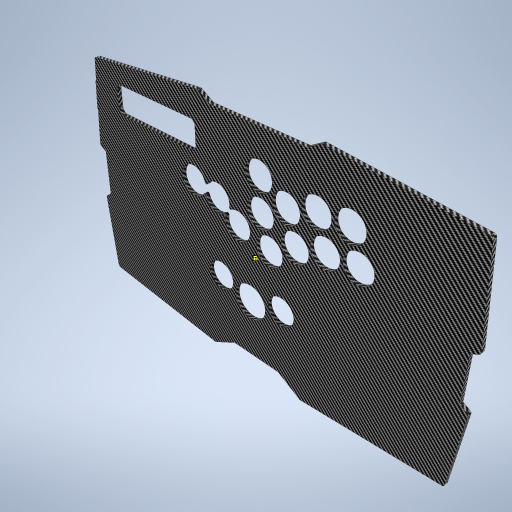
# Autodesk Inventor part: Top_Plate
Saved by Autodesk Inventor 2024 (Build 280153000, 153)
## iProperties
Created: 2023-09-20
Part Number: Top_Plate
Material: 常规
Document SubType Name: Modeling
Designer: nicx5
Density: 1 g/cm^3
Appearance: 碳纤维
Author: nicx5
Autodesk Inventor part; units mm, degrees
ref_plane "YZ Plane" through (0, 0, 0) normal (1, 0, 0) x (0, 1, 0)
ref_plane "XZ Plane" through (0, 0, 0) normal (0, 1, 0) x (-1, 0, 0)
derived "Frame.ipt"
sketch "top面板草图" plane through (0, 0, -3) normal (0, 0, 1) x (1, 0, 0)
  line L0 (-129.5, 55) -> (-52.5, 55)
  line L1 (-52.5, 55) -> (-52.5, 76.5)
  line L2 (-129.5, 76.5) -> (-52.5, 76.5)
  line L3 (-129.5, 55) -> (-129.5, 76.5)
  circle A0 centre (-55.7514, 33.4183) radius 11.5
  circle A1 centre (-34.0856, 29.598) radius 11.5
  circle A2 centre (-16.0643, 16.9793) radius 11.5
  circle A3 centre (-32.1234, -29.7121) radius 11.5
  circle A4 centre (-5.0643, -36.9094) radius 14.5
  circle A5 centre (21.9949, -29.7121) radius 11.5
  circle A6 centre (11.4783, 10.9768) radius 11.5
  circle A7 centre (3.7009, 34.6338) radius 11.5
  circle A8 centre (2.0127, 59.4994) radius 11.5
  circle A9 centre (24.0951, 47.2859) radius 11.5
  circle A10 centre (31.8725, 23.629) radius 11.5
  circle A11 centre (54.6939, 31.0574) radius 11.5
  circle A12 centre (46.9166, 54.7144) radius 11.5
  circle A13 centre (70.8507, 56.4914) radius 11.5
  circle A14 centre (78.628, 32.8344) radius 11.5
  line L4 (157.6336, 21.2378) -> (151.7356, 88.6532)
  line L5 (151.7356, 88.6532) -> (48.367, 97.6967)
  line L6 (48.367, 97.6967) -> (38.067, 91.75)
  line L7 (38.067, 91.75) -> (-38.067, 91.75)
  line L8 (-38.067, 91.75) -> (-48.367, 97.6967)
  line L9 (-48.367, 97.6967) -> (-151.7356, 88.6532)
  line L10 (-151.7356, 88.6532) -> (-153.2586, 71.2446)
  line L11 (-153.2586, 71.2446) -> (-154.5006, 70.2025)
  line L12 (157.6336, 21.2378) -> (151.75, 17.8409)
  line L13 (151.75, -17.8409) -> (157.6336, -21.2378)
  line L14 (157.6336, -21.2378) -> (152.1781, -83.5953)
  line L15 (-20.7465, -81.75) -> (20.7465, -81.75)
  line L16 (20.7465, -81.75) -> (40.8177, -93.3381)
  line L17 (40.8177, -93.3381) -> (152.1781, -83.5953)
  line L18 (-157.6336, -21.2378) -> (-152.1781, -83.5953)
  line L19 (-152.1781, -83.5953) -> (-40.8177, -93.3381)
  line L20 (-40.8177, -93.3381) -> (-20.7465, -81.75)
  line L21 (-157.6336, -21.2378) -> (-151.7501, -17.841)
  line L22 (-151.7501, 17.841) -> (-157.6336, 21.2378)
  line L23 (-157.6336, 21.2378) -> (-155.158, 49.5347)
  line L24 (-155.158, 49.5347) -> (-156.2001, 50.7767)
  line L25 (-154.5006, 70.2025) -> (-155.6, 70.2986)
  line L26 (-156.2001, 50.7767) -> (-157.2995, 50.8728)
  line L27 (-155.6, 70.2986) -> (-157.2995, 50.8728)
  line L28 (-151.7501, -17.841) -> (-151.7501, 17.841)
  line L29 (151.75, 17.8409) -> (151.75, -17.8409)
  point P0 (0, 0)
  point P1 (-154.577, 70.4647)
  point P2 (-156.3209, 50.5317)
  point P3 (-26.9988, 20.5412)
  point P4 (-45.5009, 28.205)
  point P5 (-44.3361, 34.8113)
  point P6 (-23.1511, 26.0362)
  dimension "d6" = 23
  measures "d6" diameter of A10
ref_plane "工作平面1" through (-151.7501, -17.841, -3) normal (0, 0, -1) x (0, 1, 0)
sketch "草图2" plane through (-151.7501, -17.841, -3) normal (0, 0, -1) x (0, 1, 0)
  line L0 (106.4941, 0.0146) -> (89.0856, -1.5085)
  line L1 (89.0856, -1.5085) -> (88.0434, -2.7505)
  line L2 (88.0434, -2.7505) -> (88.1396, -3.8498)
  line L3 (88.1396, -3.8498) -> (68.7138, -5.5494)
  line L4 (68.6176, -4.45) -> (68.7138, -5.5494)
  line L5 (67.3756, -3.4079) -> (68.6176, -4.45)
  line L6 (39.0788, -5.8835) -> (67.3756, -3.4079)
  line L7 (35.6819, 0) -> (39.0788, -5.8835)
  line L8 (0, 0) -> (35.6819, 0)
  line L9 (-3.3968, -5.8835) -> (0, 0)
  line L10 (-3.3968, -5.8835) -> (-65.7544, -0.4279)
  line L11 (-65.7544, -0.4279) -> (-75.4972, 110.9324)
  line L12 (-75.4972, 110.9324) -> (-63.909, 131.0036)
  line L13 (-63.909, 131.0036) -> (-63.909, 172.4966)
  line L14 (-63.909, 172.4966) -> (-75.4972, 192.5678)
  line L15 (-75.4972, 192.5678) -> (-65.7544, 303.9282)
  line L16 (-3.3968, 309.3837) -> (-65.7544, 303.9282)
  line L17 (0.0001, 303.5001) -> (-3.3968, 309.3837)
  line L18 (35.6819, 303.5001) -> (0.0001, 303.5001)
  line L19 (39.0788, 309.3837) -> (35.6819, 303.5001)
  line L20 (39.0788, 309.3837) -> (106.4941, 303.4857)
  line L21 (106.4941, 303.4857) -> (115.5377, 200.1171)
  line L22 (115.5377, 200.1171) -> (109.591, 189.8171)
  line L23 (109.591, 189.8171) -> (109.591, 113.6831)
  line L24 (109.591, 113.6831) -> (115.5377, 103.3831)
  line L25 (115.5377, 103.3831) -> (106.4941, 0.0146)
  line L26 (94.341, 22.2501) -> (94.341, 99.2501)
  line L27 (72.841, 22.2501) -> (94.341, 22.2501)
  line L28 (72.841, 99.2501) -> (94.341, 99.2501)
  line L29 (72.841, 22.2501) -> (72.841, 99.2501)
  arc A0 (45.2153, 105.1895) -> (53.7952, 106.7024) centre (51.2592, 95.9987) ccw
  arc A1 (44.1821, 129.9104) -> (37.0455, 124.9133) centre (34.8203, 135.6858) ccw
  circle A2 centre (-11.8711, 119.6267) radius 11
  circle A3 centre (-19.0685, 146.6858) radius 13.5
  circle A4 centre (-11.8711, 173.745) radius 11
  circle A5 centre (28.8178, 163.2284) radius 11
  circle A6 centre (52.4748, 155.451) radius 11
  circle A7 centre (77.3404, 153.7629) radius 11
  circle A8 centre (65.1269, 175.8453) radius 11
  circle A9 centre (41.4699, 183.6226) radius 11
  circle A10 centre (48.8984, 206.444) radius 11
  circle A11 centre (72.5554, 198.6667) radius 11
  circle A12 centre (74.3324, 222.6008) radius 11
  circle A13 centre (50.6754, 230.3782) radius 11
  line L30 (44.4988, 128.7211) -> (44.2045, 129.1414)
  line L31 (38.0548, 124.209) -> (37.7605, 124.6292)
  line L32 (53.2672, 107.262) -> (53.1781, 107.7672)
  line L33 (45.5201, 105.896) -> (45.431, 106.4012)
  arc A14 (38.0771, 123.4399) -> (44.903, 106.9608) centre (47.439, 117.6645) ccw
  arc A15 (53.4829, 108.4737) -> (45.2138, 128.4371) centre (47.439, 117.6645) ccw
  arc A16 (44.4988, 128.7211) -> (45.2138, 128.4371) centre (45.0722, 129.1226) ccw
  arc A17 (44.1821, 129.9104) -> (44.2045, 129.1414) centre (44.7779, 129.5429) ccw
  arc A18 (38.0771, 123.4399) -> (38.0548, 124.209) centre (37.4814, 123.8075) ccw
  arc A19 (37.7605, 124.6292) -> (37.0455, 124.9133) centre (37.1871, 124.2277) ccw
  arc A20 (53.2672, 107.262) -> (53.7952, 106.7024) centre (53.9566, 107.3835) ccw
  arc A21 (53.4829, 108.4737) -> (53.1781, 107.7672) centre (53.8675, 107.8888) ccw
  arc A22 (45.431, 106.4012) -> (44.903, 106.9608) centre (44.7416, 106.2797) ccw
  arc A23 (45.2153, 105.1895) -> (45.5201, 105.896) centre (44.8307, 105.7744) ccw
  point P0 (17.841, 151.7501)
  point P1 (38.3248, 123.8234)
  point P2 (37.4905, 125.0148)
  point P3 (53.349, 106.7984)
  point P4 (45.6018, 105.4324)
  point P5 (45.3492, 106.8648)
  point P6 (44.7688, 128.3355)
  point P7 (43.9345, 129.527)
  point P8 (53.0964, 108.2308)
  dimension "d7" = 22
  dimension "d8" = 22
  dimension "d9" = 22
  dimension "d10" = 22
  dimension "d11" = 22
  dimension "d12" = 22
  dimension "d13" = 22
  dimension "d14" = 22
  dimension "d15" = 22
  dimension "d16" = 22
  dimension "d17" = 27
  dimension "d18" = 22
  dimension "d19" = 22
  dimension "d21" = 22
  dimension "d24" = 0.7
  dimension "d25" = 0.7
  constraints: 68 end point, 32 point on circle, 24 centre point, 16 tangent, 8 point on line, 6 equal radius
  measures "d7" diameter of A6
  measures "d8" diameter of A5
  measures "d9" diameter of A9
  measures "d10" diameter of A10
  measures "d11" diameter of A13
  measures "d12" diameter of A12
  measures "d13" diameter of A11
  measures "d14" diameter of A8
  measures "d15" diameter of A7
  measures "d16" diameter of A4
  measures "d17" diameter of A3
  measures "d18" diameter of A2
  measures "d19" diameter of A1
  measures "d21" diameter of A0
  measures "d24" radius of A16
  measures "d25" radius of A20
extrude "拉伸3" add sketch "草图2" along normal blind 3
fillet "圆角2" radius 2 12 edges at (-151.7356, 88.6532, -4.5) (-48.367, 97.6967, -4.5) (48.367, 97.6967, -4.5) (151.7356, 88.6532, -4.5) (157.6336, 21.2378, -4.5) (157.6336, -21.2378, -4.5) (152.1781, -83.5953, -4.5) (40.8177, -93.3381, -4.5) (-40.8177, -93.3381, -4.5) (-152.1781, -83.5953, -4.5) (-157.6336, -21.2378, -4.5) (-157.6336, 21.2378, -4.5)
fillet "圆角3" radius 2 1 edges at (-156.4497, 60.5857, -3)
fillet "圆角4" radius 4 4 edges at (-129.5, 76.5, -4.5) (-129.5, 55, -4.5) (-52.5, 76.5, -4.5) (-52.5, 55, -4.5)
